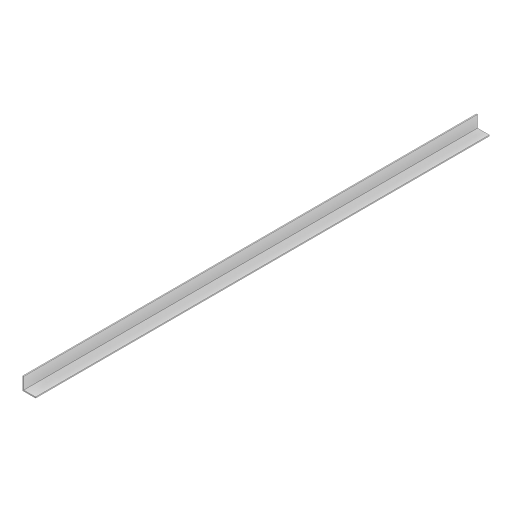
# Autodesk Inventor part: GUIA_CANALETA
Saved by Autodesk Inventor 2024 (Build 280153000, 153)
## iProperties
Created: 2024-08-15
Part Number: GUIA_CANALETA
Material: Generic
Document SubType Name: Modeling
Designer: Jhuliams
Density: 1 g/cm^3
Appearance: Default
Author: Jhuliams
Autodesk Inventor part; units mm, degrees
ref_plane "YZ Plane" through (0, 0, 0) normal (1, 0, 0) x (0, 1, 0)
ref_plane "XZ Plane" through (0, 0, 0) normal (0, 1, 0) x (-1, 0, 0)
ref_plane "XY Plane" through (0, 0, 0) normal (0, 0, 1) x (1, 0, 0)
sketch "Sketch2" plane through (0, 0, 0) normal (0, 0, 1) x (1, 0, 0)
  line L0 (0, 0) -> (1.5, 0)
  line L1 (1.5, 0) -> (1.5, 19)
  line L2 (1.5, 19) -> (0, 19)
  line L3 (0, 19) -> (0, 0)
  line L4 (0, 0) -> (19, 0)
  line L5 (19, 0) -> (19, 1.5)
  line L6 (19, 1.5) -> (0, 1.5)
  line L7 (0, 1.5) -> (0, 0)
  point P0 (1.5, 1.5)
  dimension "d0" = 1.5
  dimension "d1" = 19
  dimension "d2" = 19
  dimension "d3" = 1.5
  constraints: 16 end point, 4 parallel, 2 horizontal, 2 perpendicular
  measures "d0" distance of L2.end L1.end
  measures "d1" distance of L1.end L0.end
  measures "d2" distance of L6.end L5.end
  measures "d3" distance of L5.end L4.end
extrude "Extrusion1" add sketch "Sketch2" along normal mid plane 670
body "Solid1"
